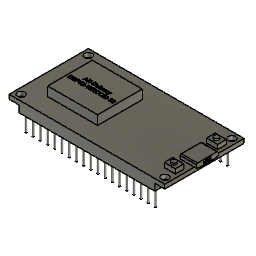
ESP32_v1 (Autodesk Fusion 360 design; units mm, degrees)
Autodesk Fusion 360 part; units mm, degrees
sketch "Skizze1" plane through (0, 0, 0) normal (0, 0, 1) x (1, 0, 0) in component "ESP32"
  line L0 (0, 0) -> (55, 0)
  line L1 (55, 0) -> (55, 28)
  line L2 (55, 28) -> (0, 28)
  line L3 (0, 28) -> (0, 0)
  circle A0 centre (2.1, 2.15) radius 1.3
  circle A1 centre (2.1, 25.85) radius 1.3
  circle A2 centre (52.9, 25.85) radius 1.3
  circle A3 centre (52.9, 2.15) radius 1.3
  dimension "d7" = 55
  dimension "d8" = 28
  dimension "d9" = 2.6
  dimension "d10" = 2.6
  dimension "d11" = 2.6
  dimension "d12" = 2.6
  constraint horizontal L0
  constraint vertical L1
  constraint horizontal L2
  constraint vertical L3
  constraint coincident L0.start L3.end
  measures "d7" distance of L0.start L0.end
  measures "d8" distance of L0.start L2.end
  measures "d9" diameter of A0
  measures "d10" diameter of A1
  measures "d11" diameter of A3
  measures "d12" diameter of A2
extrude "Extrusion2" add sketch "Skizze1" along normal blind 1.5 in component "ESP32"
sketch "Skizze3" plane through (0, 0, 1.5) normal (0, 0, 1) x (-1, 0, 0) in component "ESP32"
  circle A0 centre (-2.1, -25.85) radius 1.3
  circle A1 centre (-52.9, -2.15) radius 1.3
  circle A2 centre (-52.9, -25.85) radius 1.3
  circle A3 centre (-2.1, -2.15) radius 1.3
  line L0 (0, -28) -> (0, 0)
  line L1 (0, 0) -> (-55, 0)
  line L2 (-55, 0) -> (-55, -28)
  line L3 (-55, -28) -> (0, -28)
  line L4 (-7.5, -21.875) -> (-25.15, -21.875)
  line L5 (-25.15, -21.875) -> (-25.15, -6.125)
  line L6 (-25.15, -6.125) -> (-7.5, -6.125)
  line L7 (-7.5, -6.125) -> (-7.5, -21.875)
  dimension "d17" = 17.65
  dimension "d18" = 15.75
  constraint horizontal L4
  constraint vertical L5
  constraint horizontal L6
  constraint vertical L7
  measures "d17" distance of L4.start L4.end
  measures "d18" distance of L4.start L6.end
extrude "Extrusion3" add sketch "Skizze3" along normal blind 3.25 contours L4 L5 L6 L7 in component "ESP32"
sketch "Skizze4" plane through (0, 0, 1.5) normal (0, 0, 1) x (-1, 0, 0) in component "ESP32"
  line L0 (-7.5, -6.125) -> (-7.5, -21.875)
  line L1 (-7.5, -21.875) -> (-25.15, -21.875)
  line L2 (-25.15, -21.875) -> (-25.15, -6.125)
  line L3 (-25.15, -6.125) -> (-7.5, -6.125)
  circle A0 centre (-2.1, -25.85) radius 1.3
  circle A1 centre (-52.9, -2.15) radius 1.3
  circle A2 centre (-52.9, -25.85) radius 1.3
  circle A3 centre (-2.1, -2.15) radius 1.3
  line L4 (0, -28) -> (0, 0)
  line L5 (0, 0) -> (-55, 0)
  line L6 (-55, 0) -> (-55, -28)
  line L7 (-55, -28) -> (0, -28)
  line L8 (-56, -17.875) -> (-50.3, -17.875)
  line L9 (-50.3, -17.875) -> (-50.3, -10.125)
  line L10 (-50.3, -10.125) -> (-56, -10.125)
  line L11 (-56, -10.125) -> (-56, -17.875)
  line L12 (-7.5, -6.125) -> (-25.15, -6.125) construction
  line L13 (-25.15, -6.125) -> (-25.15, -21.875) construction
  line L14 (-25.15, -21.875) -> (-7.5, -21.875) construction
  line L15 (-7.5, -21.875) -> (-7.5, -6.125) construction
  dimension "d21" = 5.7
  dimension "d22" = 7.75
  text T0 "AZ-Delivery\nESP32-WROOM-32" font "Arial" height 1.3 align centre middle in box 17.65 x 15.75 at (-7.5, -6.125) x (-1, 0) y (0, -1) spacing 1
  constraint horizontal L8
  constraint vertical L9
  constraint horizontal L10
  constraint vertical L11
  constraint coincident L2.end
  constraint coincident L0.end
  measures "d21" distance of L8.start L8.end
  measures "d22" distance of L8.start L10.end
extrude "Extrusion4" add sketch "Skizze4" along normal blind 1.7 contours L6 L8 L10 L11 | L6 L8 L9 L10 in component "ESP32"
sketch "Skizze5" plane through (56, 0, 0) normal (1, 0, 0) x (0, 1, 0) in component "ESP32"
  line L0 (10.125, 1.5) -> (17.875, 1.5)
  line L1 (17.875, 1.5) -> (17.875, 3.2)
  line L2 (17.875, 3.2) -> (10.125, 3.2)
  line L3 (10.125, 3.2) -> (10.125, 1.5)
  line L4 (11.3, 1.5) -> (16.7, 1.5)
  line L5 (10.55, 3.2) -> (17.45, 3.2)
  line L6 (10.125, 2.92) -> (10.125, 1.82)
  line L7 (17.875, 2.92) -> (17.875, 1.82)
  line L8 (10.125, 2.92) -> (10.55, 3.2)
  line L9 (17.45, 3.2) -> (17.875, 2.92)
  line L10 (17.875, 1.82) -> (16.7, 1.5)
  line L11 (11.3, 1.5) -> (10.125, 1.82)
  line L12 (11.3128, 1.5) -> (16.7, 1.5) construction
  line L13 (16.7, 1.5) -> (16.7, 3.2) construction
  line L14 (16.7, 3.2) -> (11.3128, 3.2) construction
  line L15 (11.3128, 3.2) -> (11.3128, 1.5) construction
  dimension "d26" = 5.4
  dimension "d27" = 6.9
  dimension "d28" = 1.1
  dimension "d29" = 1.1
  text T0 "USB" font "Arial" height 1 align centre middle in box 5.3872 x 1.7 at (11.3128, 1.5) x (1, 0) y (0, 1) spacing 1
  constraint horizontal L4
  constraint midpoint L0 L4
  constraint horizontal L5
  constraint midpoint L2 L5
  constraint vertical L6
  constraint vertical L7
  constraint coincident L2
  constraint coincident L4.end
  measures "d26" distance of L4.start L4.end
  measures "d27" distance of L5.start L5.end
  measures "d28" distance of L6.start L6.end
  measures "d29" distance of L7.start L7.end
extrude "Extrusion5" cut sketch "Skizze5" against normal blind 6 contours L2 L3 L8 in component "ESP32"
extrude "Extrusion6" cut sketch "Skizze5" against normal blind 6 contours L0 L3 L11 | L0 L1 L10 | L1 L2 L9 in component "ESP32"
extrude "Extrusion7" cut sketch "Skizze5" against normal blind 1 text T0 in component "ESP32"
extrude "Extrusion8" cut sketch "Skizze4" along normal blind 9 text T0 in component "ESP32"
sketch "Skizze6" plane through (0, 0, 0) normal (0, 0, -1) x (1, 0, 0) in component "ESP32"
  circle A0 centre (2.1, -25.85) radius 1.3
  circle A1 centre (52.9, -2.15) radius 1.3
  circle A2 centre (52.9, -25.85) radius 1.3
  circle A3 centre (2.1, -2.15) radius 1.3
  line L0 (0, 0) -> (0, -28)
  line L1 (0, -28) -> (55, -28)
  line L2 (55, -28) -> (55, 0)
  line L3 (55, 0) -> (0, 0)
  line L4 (3.5, 0) -> (51.5, 0)
  line L5 (51.5, 0) -> (51.5, -2.5)
  line L6 (51.5, -2.5) -> (3.5, -2.5)
  line L7 (3.5, -2.5) -> (3.5, 0)
  line L8 (3.5, -25.5) -> (51.5, -25.5)
  line L9 (51.5, -28) -> (3.5, -28)
  line L10 (51.5, -25.5) -> (51.5, -28)
  line L11 (3.5, -28) -> (3.5, -25.5)
  dimension "d38" = 48
  dimension "d39" = 2.5
  dimension "d40" = 48
  dimension "d41" = 2.5
  constraint horizontal L4
  constraint vertical L5
  constraint horizontal L6
  constraint vertical L7
  constraint midpoint L3 L4
  constraint horizontal L8
  constraint vertical L10
  constraint horizontal L9
  constraint vertical L11
  measures "d38" distance of L4.start L4.end
  measures "d39" distance of L4.start L6.end
  measures "d40" distance of L8.start L8.end
  measures "d41" distance of L8.start L9.end
extrude "Extrusion9" add sketch "Skizze6" along normal blind 2.4 contours L3 L4 L5 L6 L7 | L1 L8 L9 L10 L11 in component "ESP32"
sketch "Skizze7" plane through (0, 0, -2.4) normal (0, 0, -1) x (1, 0, 0) in component "ESP32"
  line L0 (3.5, -2.5) -> (51.5, -2.5)
  line L1 (51.5, -2.5) -> (51.5, 0)
  line L2 (51.5, 0) -> (3.5, 0)
  line L3 (3.5, 0) -> (3.5, -2.5)
  circle A0 centre (4.75, -1.25) radius 0.315
  circle A1 centre (7.29, -1.25) radius 0.315
  circle A2 centre (9.83, -1.25) radius 0.315
  circle A3 centre (12.37, -1.25) radius 0.315
  circle A4 centre (14.91, -1.25) radius 0.315
  circle A5 centre (17.45, -1.25) radius 0.315
  circle A6 centre (19.99, -1.25) radius 0.315
  circle A7 centre (22.53, -1.25) radius 0.315
  circle A8 centre (25.07, -1.25) radius 0.315
  circle A9 centre (27.61, -1.25) radius 0.315
  circle A10 centre (30.15, -1.25) radius 0.315
  circle A11 centre (32.69, -1.25) radius 0.315
  circle A12 centre (35.23, -1.25) radius 0.315
  circle A13 centre (37.77, -1.25) radius 0.315
  circle A14 centre (40.31, -1.25) radius 0.315
  circle A15 centre (42.85, -1.25) radius 0.315
  circle A16 centre (45.39, -1.25) radius 0.315
  circle A17 centre (47.93, -1.25) radius 0.315
  circle A18 centre (50.47, -1.25) radius 0.315
  circle A19 centre (17.45, -26.75) radius 0.315
  circle A20 centre (40.31, -26.75) radius 0.315
  circle A21 centre (9.83, -26.75) radius 0.315
  circle A22 centre (35.23, -26.75) radius 0.315
  circle A23 centre (27.61, -26.75) radius 0.315
  circle A24 centre (30.15, -26.75) radius 0.315
  circle A25 centre (25.07, -26.75) radius 0.315
  circle A26 centre (22.53, -26.75) radius 0.315
  circle A27 centre (4.75, -26.75) radius 0.315
  circle A28 centre (47.93, -26.75) radius 0.315
  circle A29 centre (42.85, -26.75) radius 0.315
  circle A30 centre (32.69, -26.75) radius 0.315
  circle A31 centre (7.29, -26.75) radius 0.315
  circle A32 centre (37.77, -26.75) radius 0.315
  circle A33 centre (45.39, -26.75) radius 0.315
  circle A34 centre (12.37, -26.75) radius 0.315
  circle A35 centre (50.47, -26.75) radius 0.315
  circle A36 centre (14.91, -26.75) radius 0.315
  circle A37 centre (19.99, -26.75) radius 0.315
  dimension "d44" = 0.63
  dimension "d47" = 2.54
  dimension "d48" = 0
  dimension "d51" = 2.54
  dimension "d52" = 0
  dimension "d53" = 0.63
  measures "d44" diameter of A0
  measures "d53" diameter of A27
extrude "Extrusion10" add sketch "Skizze7" along normal blind 5.95 contours A0 | A1 | A2 | A3 | A4 | A5 | A6 | A7 | A8 | A9 | A10 | A11 | A12 | A13 | A14 | A15 | A16 | A17 | A18 | A19 | A20 | A21 | A22 | A23 | A24 | A25 | A26 | A27 | A28 | A29 | A30 | A31 | A32 | A33 | A34 | A35 | A36 | A37 in component "ESP32"
sketch "Skizze8" plane through (0, 0, 1.5) normal (0, 0, 1) x (-1, 0, 0) in component "ESP32"
  circle A0 centre (-2.1, -2.15) radius 1.3
  circle A1 centre (-52.9, -25.85) radius 1.3
  circle A2 centre (-52.9, -2.15) radius 1.3
  circle A3 centre (-2.1, -25.85) radius 1.3
  line L0 (-7.5, -6.125) -> (-7.5, -21.875)
  line L1 (-7.5, -21.875) -> (-25.15, -21.875)
  line L2 (-25.15, -21.875) -> (-25.15, -6.125)
  line L3 (-25.15, -6.125) -> (-7.5, -6.125)
  line L4 (-50.3, -11.3) -> (-50.3, -16.7)
  line L5 (-50.3, -16.7) -> (-55, -16.7)
  line L6 (-55, -16.7) -> (-55, -28)
  line L7 (-55, -28) -> (0, -28)
  line L8 (0, -28) -> (0, 0)
  line L9 (0, 0) -> (-55, 0)
  line L10 (-55, 0) -> (-55, -11.3)
  line L11 (-55, -11.3) -> (-50.3, -11.3)
  line L12 (-49.85, -8) -> (-53.75, -8)
  line L13 (-53.75, -8) -> (-53.75, -5)
  line L14 (-53.75, -5) -> (-49.85, -5)
  line L15 (-49.85, -5) -> (-49.85, -8)
  circle A4 centre (-51.8, -6.5) radius 0.875
  line L16 (-53.75, -22.95) -> (-53.75, -19.95)
  circle A5 centre (-51.8, -21.45) radius 0.875
  line L17 (-53.75, -19.95) -> (-49.85, -19.95)
  line L18 (-49.85, -19.95) -> (-49.85, -22.95)
  line L19 (-49.85, -22.95) -> (-53.75, -22.95)
  dimension "d56" = 3.9
  dimension "d57" = 3
  dimension "d58" = 1.75
  dimension "d59" = 3.9
  dimension "d60" = 3
  dimension "d61" = 1.75
  constraint horizontal L12
  constraint vertical L13
  constraint horizontal L14
  constraint vertical L15
  constraint horizontal L19
  constraint vertical L16
  constraint horizontal L17
  constraint vertical L18
  measures "d56" distance of L12.start L12.end
  measures "d57" distance of L12.start L14.end
  measures "d58" diameter of A4
  measures "d59" distance of L16.start L18.end
  measures "d60" distance of L18.end L17.end
  measures "d61" diameter of A5
extrude "Extrusion11" add sketch "Skizze8" along normal blind 1.6 contours L12 L13 L14 L15 | A4 | L16 L17 L18 L19 | A5 in component "ESP32"
extrude "Extrusion12" add sketch "Skizze8" along normal blind 2.2 contours A4 | A5 in component "ESP32"
component "ESP32" placed x (1, 0, 0) y (0, 1, 0) z (0, 0, 1) at (0, 0, 0)
equation "d19 = 4.75 mm - 1.5 mm"
equation "d23 = 4.2 mm - 2.5 mm"
equation "d47 = 1.9 mm + 0.64 mm"
equation "d62 = 3.1 mm - 1.5 mm"
equation "d64 = 3.7 mm - 1.5 mm"
